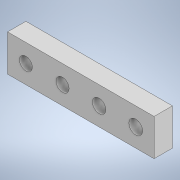
# Autodesk Inventor part: Hole-Gauge
Saved by Autodesk Inventor 2022 (Build 260153000, 153)
## iProperties
Created: 2024-07-11
Part Number: Hole-Gauge
Material: 一般
Document SubType Name: Modeling
Designer: yamashita1
Density: 1 g/cm^3
Appearance: 既定
Author: yamashita1
Autodesk Inventor part; units mm, degrees
ref_plane "YZ Plane" through (0, 0, 0) normal (1, 0, 0) x (0, 1, 0)
ref_plane "XZ Plane" through (0, 0, 0) normal (0, 1, 0) x (-1, 0, 0)
ref_plane "XY Plane" through (0, 0, 0) normal (0, 0, 1) x (1, 0, 0)
sketch "スケッチ1" plane through (0, 0, 0) normal (0, 0, 1) x (1, 0, 0)
  line L0 (-12, 3) -> (12, 3)
  line L1 (12, 3) -> (12, -3)
  line L2 (12, -3) -> (-12, -3)
  line L3 (-12, -3) -> (-12, 3)
  point P0 (0, 0)
  point P1 (-12, 0)
  point P2 (0, 3)
  dimension "d0" = 24
  dimension "d1" = 6
  constraints: 8 end point, 2 midpoint, 2 parallel, 1 horizontal, 1 horizontal alignment, 1 perpendicular, 1 vertical alignment
  measures "d0" distance of L1.end L2.end
  measures "d1" distance of L0.end L1.end
extrude "押し出し1" add sketch "スケッチ1" along normal blind 3
sketch "スケッチ2" plane through (0, 0, 3) normal (0, 0, 1) x (1, 0, 0)
  circle A0 centre (-9, 0) radius 1.05
  circle A1 centre (-3, 0) radius 1.075
  circle A2 centre (3, 0) radius 1.1
  circle A3 centre (9, 0) radius 1.125
  line L0 (-12, 3) -> (-12, -3) projected
  point P0 (0, 0)
  dimension "d4" = 6
  dimension "d5" = 6
  dimension "d6" = 6
  dimension "d7" = 2.1
  dimension "d8" = 2.15
  dimension "d9" = 2.2
  dimension "d10" = 2.25
  dimension "d11" = 3
  constraints: 4 centre point, 4 horizontal alignment
  measures "d4" distance of A1.centre A0.centre
  measures "d5" distance of A2.centre A1.centre
  measures "d6" distance of A3.centre A2.centre
  measures "d7" diameter of A0
  measures "d8" diameter of A1
  measures "d9" diameter of A2
  measures "d10" diameter of A3
  measures "d11" distance from line of L0 A0.centre
extrude "押し出し2" cut sketch "スケッチ2" against normal through all
equation "\"d5\" = d4"
equation "\"d6\" = d4"
